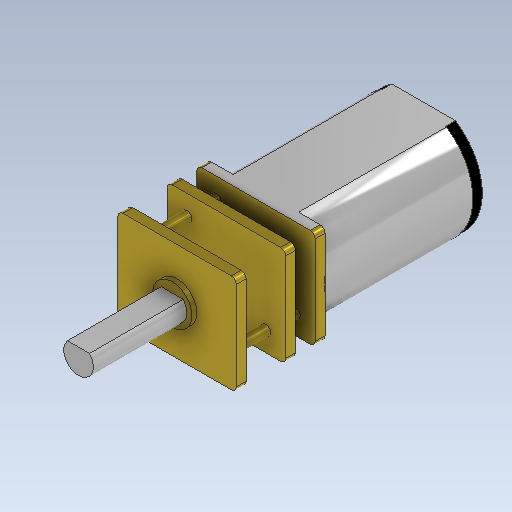
# Autodesk Inventor part: minimotor
Saved by Autodesk Inventor 2020.2 (Build 242310000, 310)
## iProperties
Created: 2019-10-27
Part Number: minimotor
Material: Generic
Document SubType Name: Modeling
Designer: 19Bar
Density: 1 g/cm^3
Appearance: Default
Author: 19Bar
Autodesk Inventor part; units mm, degrees
ref_plane "YZ Plane" through (0, 0, 0) normal (1, 0, 0) x (0, 1, 0)
ref_plane "XZ Plane" through (0, 0, 0) normal (0, 1, 0) x (-1, 0, 0)
ref_plane "XY Plane" through (0, 0, 0) normal (0, 0, 1) x (1, 0, 0)
sketch "Sketch1" plane through (0, 0, 0) normal (0, 0, 1) x (1, 0, 0)
  circle A0 centre (0, 0) radius 6
  line L0 (0, 0) -> (0, 5)
  line L1 (0, 5) -> (3.3166, 5)
  line L2 (0, 5) -> (-3.3166, 5)
  line L3 (0, 0) -> (0, -5)
  line L4 (0, -5) -> (3.3166, -5)
  line L5 (0, -5) -> (-3.3166, -5)
  dimension "d0" = 12
  dimension "d1" = 5
  dimension "d2" = 5
  constraints: 12 end point, 4 point on circle, 3 point on line, 2 perpendicular, 1 centre point, 1 coincident, 1 vertical
  measures "d0" diameter of A0
  measures "d1" distance of L0.start L0.end
  measures "d2" distance of L0.start L3.end
extrude "Extrusion1" add sketch "Sketch1" along normal blind 15 contours A0 L4 L3 L0 L1 | L2 L0 L3 L5 A0
sketch "Sketch2" plane through (0, 0, 15) normal (0, 0, 1) x (1, 0, 0)
  arc A0 (-3.3166, 5) -> (-3.3166, -5) centre (0, 0) ccw projected
  line L0 (-6, 0) -> (-6, 4.5)
  line L1 (-5.5, 5) -> (5.5, 5)
  line L2 (6, 4.5) -> (6, -4.5)
  line L3 (5.5, -5) -> (-5.5, -5)
  line L4 (-6, -4.5) -> (-6, 5)
  arc A1 (-5.5, 5) -> (-6, 4.5) centre (-5.5, 4.5) ccw
  arc A2 (-6, -4.5) -> (-5.5, -5) centre (-5.5, -4.5) ccw
  arc A3 (5.5, -5) -> (6, -4.5) centre (5.5, -4.5) ccw
  arc A4 (6, 4.5) -> (5.5, 5) centre (5.5, 4.5) ccw
  point P0 (6, -5)
  point P1 (-6, -5)
  dimension "d5" = 12
  dimension "d6" = 0.5
  dimension "d32" = 10
  dimension "d33" = 5
  constraints: 10 end point, 9 point on circle, 9 tangent, 6 point on line, 4 centre point, 3 equal radius, 2 parallel, 1 horizontal, 1 perpendicular, 1 vertical
  measures "d5" distance of point (6, -5) point (-6, -5)
  measures "d6" radius of A1
  measures "d32" distance between parallel lines of L1 L3
  measures "d33" distance from line of point (0, 0) L3
extrude "Extrusion2" add sketch "Sketch2" along normal blind 1
sketch "Sketch3" plane through (0, 0, 16) normal (0, 0, 1) x (1, 0, 0)
  line L0 (0, 0) -> (-4, 0)
  line L1 (-4, 0) -> (-4, 3)
  line L2 (0, 0) -> (0, -3)
  line L3 (0, -3) -> (4, -3)
  circle A0 centre (-4, 3) radius 0.5
  circle A1 centre (4, -3) radius 0.5
  dimension "d9" = 4
  dimension "d10" = 3
  dimension "d11" = 3
  dimension "d12" = 4
  dimension "d13" = 1
  dimension "d14" = 1
  constraints: 8 end point, 2 centre point, 2 coincident, 2 horizontal, 1 perpendicular, 1 vertical
  measures "d9" distance of L0.start L0.end
  measures "d10" distance of L0.end L1.end
  measures "d11" distance of L0.start L2.end
  measures "d12" distance of L2.end L3.end
  measures "d13" diameter of A0
  measures "d14" diameter of A1
extrude "Extrusion3" add sketch "Sketch3" along normal blind 2
sketch "Sketch4" plane through (-4, 3, 18) normal (0, 0, 1) x (1, 0, 0)
  line L0 (-1.5, 2) -> (9.5, 2)
  line L1 (10, 1.5) -> (10, -7.5)
  line L2 (9.5, -8) -> (-1.5, -8)
  line L3 (-2, -7.5) -> (-2, 1.5)
  arc A0 (-1.5, 2) -> (-2, 1.5) centre (-1.5, 1.5) ccw
  arc A1 (-2, -7.5) -> (-1.5, -8) centre (-1.5, -7.5) ccw
  arc A2 (9.5, -8) -> (10, -7.5) centre (9.5, -7.5) ccw
  arc A3 (10, 1.5) -> (9.5, 2) centre (9.5, 1.5) ccw
  line L4 (-1.5, -8) -> (9.5, -8) projected
  line L5 (-2, 1.5) -> (-2, -7.5) projected
  point P0 (4, -3)
  dimension "d17" = 0.5
  dimension "d36" = 10
  dimension "d37" = 12
  dimension "d38" = 0
  dimension "d39" = 0
  constraints: 8 end point, 8 point on circle, 8 tangent, 4 centre point, 3 equal radius, 2 parallel, 1 horizontal, 1 perpendicular
  measures "d17" radius of A0
  measures "d36" distance between parallel lines of L0 L2
  measures "d37" distance between parallel lines of L3 L1
  measures "d38" distance between parallel lines of L4 L2
  measures "d39" distance between parallel lines of L5 L3
extrude "Extrusion4" add sketch "Sketch4" along normal blind 1
sketch "Sketch5" plane through (-4, 3, 19) normal (0, 0, 1) x (1, 0, 0)
  circle A0 centre (0, 0) radius 0.5 projected
  circle A1 centre (0, 0) radius 0.5
  circle A2 centre (8, -6) radius 0.5 projected
  circle A3 centre (8, -6) radius 0.5
  point P0 (4, -3)
  point P1 (7.9, -5.5101)
  point P2 (7.9, -6.4899)
  constraints: 2 centre point, 2 coincident
extrude "Extrusion5" add sketch "Sketch5" along normal blind 4
sketch "Sketch6" plane through (-4, 3, 23) normal (0, 0, 1) x (1, 0, 0)
  line L0 (-1.5, 2) -> (9.5, 2)
  line L1 (10, 1.5) -> (10, -7.5)
  line L2 (9.5, -8) -> (-1.5, -8)
  line L3 (-2, -7.5) -> (-2, 1.5)
  arc A0 (-1.5, 2) -> (-2, 1.5) centre (-1.5, 1.5) ccw
  arc A1 (10, 1.5) -> (9.5, 2) centre (9.5, 1.5) ccw
  arc A2 (9.5, -8) -> (10, -7.5) centre (9.5, -7.5) ccw
  arc A3 (-2, -7.5) -> (-1.5, -8) centre (-1.5, -7.5) ccw
  line L4 (-1.5, -8) -> (9.5, -8) projected
  line L5 (-2, 1.5) -> (-2, -7.5) projected
  point P0 (4, -3)
  dimension "d22" = 0.5
  dimension "d40" = 10
  dimension "d41" = 12
  dimension "d42" = 0
  dimension "d43" = 0
  constraints: 8 end point, 8 point on circle, 8 tangent, 4 centre point, 3 equal radius, 2 parallel, 1 horizontal, 1 perpendicular
  measures "d22" radius of A0
  measures "d40" distance between parallel lines of L0 L2
  measures "d41" distance between parallel lines of L3 L1
  measures "d42" distance between parallel lines of L4 L2
  measures "d43" distance between parallel lines of L5 L3
extrude "Extrusion6" add sketch "Sketch6" along normal blind 1
sketch "Sketch7" plane through (-4, 3, 24) normal (0, 0, 1) x (1, 0, 0)
  circle A0 centre (4, -3) radius 1.5
  line L0 (4, -3) -> (4, -2)
  line L1 (4, -2) -> (5.118, -2)
  line L2 (4, -2) -> (2.882, -2)
  dimension "d25" = 3
  dimension "d26" = 1
  constraints: 6 end point, 2 point on circle, 1 centre point, 1 coincident, 1 perpendicular, 1 point on line, 1 vertical
  measures "d25" diameter of A0
  measures "d26" distance of L0.start L0.end
extrude "Extrusion7" add sketch "Sketch7" along normal blind 10 contours A0 L2 L1 picked at (3.9981, -3.6594)
sketch "Sketch8" plane through (0, 0, 0) normal (0, 0, -1) x (-1, 0, 0)
  circle A0 centre (0, 0) radius 5.95
  line L0 (0, 0) -> (0, -5)
  line L1 (3.3166, -5) -> (-3.3166, -5) projected
  line L2 (0, -5) -> (3.3166, -5)
  line L3 (3.3166, -5) -> (-3.2253, -5)
  line L4 (0, 0) -> (0, 5)
  line L5 (-3.3166, 5) -> (3.3166, 5) projected
  line L6 (3.289, 4.9583) -> (-3.289, 4.9583)
  point P0 (-3.2253, -5)
  point P1 (3.2253, -5)
  point P2 (3.2253, 5)
  point P3 (-3.2253, 5)
  dimension "d35" = 11.9
  dimension "d34" = 5
  constraints: 10 end point, 2 perpendicular, 1 midpoint, 1 point on line, 1 vertical, 5 other
  measures "d34" distance of L0.start L0.end
extrude "Extrusion8" add sketch "Sketch8" along normal blind 1 contours A0 L1 L0 L4 L6 | L6 L4 L5 A0 | L6 A0 L5 L4 | L4 L0 L1 A0 L6
sketch "Sketch9" plane through (0, 0, -1) normal (0, 0, -1) x (-1, 0, 0)
  arc A0 (-1.118, 1) -> (1.118, 1) centre (0, 0) ccw projected
  circle A1 centre (0, 0) radius 2.5
  dimension "d44" = 5
  constraints: 1 centre point, 1 coincident
  measures "d44" diameter of A1
extrude "Extrusion9" add sketch "Sketch9" along normal blind 0.5
sketch "Sketch10" plane through (0, 0, -1.5) normal (0, 0, -1) x (-1, 0, 0)
  circle A0 centre (0, 0) radius 0.5
  dimension "d47" = 1
  constraints: 1 centre point, 1 coincident
  measures "d47" diameter of A0
extrude "Extrusion10" add sketch "Sketch10" along normal blind 0.5
sketch "Sketch11" plane through (-4, 3, 24) normal (0, 0, 1) x (1, 0, 0)
  arc A0 (2.882, -2) -> (5.118, -2) centre (4, -3) ccw projected
  circle A1 centre (4, -3) radius 2
  dimension "d50" = 4
  constraints: 1 centre point, 1 coincident
  measures "d50" diameter of A1
extrude "Extrusion11" add sketch "Sketch11" along normal blind 0.5
body "Solid1"
